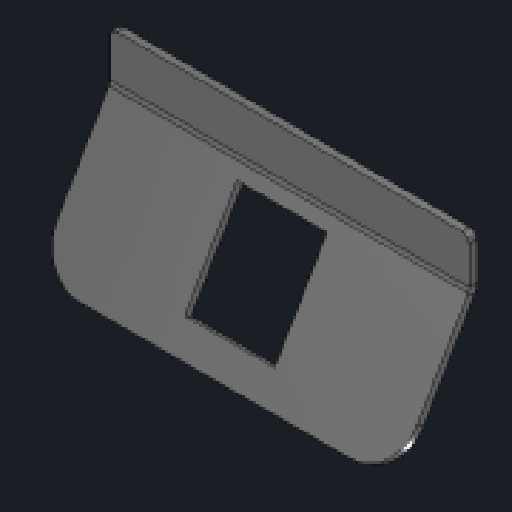
# Autodesk Inventor part: Model-4_Sheet Stifferner
Saved by Autodesk Inventor 2025.1 (Build 291241000, 241)
## iProperties
RuleStatus: InUse
Created: 2026-02-13
Part Number: Model-4_Sheet Stifferner
User Status: Released
Material: SS304
Document SubType Name: Sheet Metal
Designer: Desktop -24
Density: 7.99949 g/cm^3
Sheet Metal Rule: 1/4"
Appearance: Semi-Polished(1)
AfterDocNew0: Mat. Selection
encoded128: ÌSheet Metal (in)XÎ
Family: SS304
Author: Desktop -24
Revision Number: 0
Autodesk Inventor part; units mm, degrees
ref_plane "YZ Plane" through (0, 0, 0) normal (1, 0, 0) x (0, 1, 0)
ref_plane "XZ Plane" through (0, 0, 0) normal (0, 1, 0) x (-1, 0, 0)
ref_plane "XY Plane" through (0, 0, 0) normal (0, 0, 1) x (1, 0, 0)
sketch "Sketch1" plane through (0, 0, 0) normal (0, 0, 1) x (1, 0, 0)
  line L0 (-177.8, -19.05) -> (177.8, -19.05)
  line L1 (177.8, -19.05) -> (177.8, 19.05)
  line L2 (177.8, 19.05) -> (-177.8, 19.05)
  line L3 (-177.8, 19.05) -> (-177.8, -19.05)
  line L4 (-177.8, -19.05) -> (177.8, 19.05) construction
  line L5 (177.8, -19.05) -> (-177.8, 19.05) construction
  point P0 (0, 0)
  point P1 (0, 0)
  dimension "d31" = 355.6
  dimension "d32" = 38.1
  measures "d31" distance of L1.end L2.end
  measures "d32" distance of L0.end L1.end
extrude "Plate1" add sketch "Sketch1" along normal blind 6.35
sketch "Sketch3" plane through (177.8, -23.0251, 7.4151) normal (0, -0.5, -0.8660254) x (1, 0, 0)
  line L0 (-355.6, 0) -> (0, 0)
  line L1 (0, 0) -> (0, 125.3998)
  line L2 (0, 125.3998) -> (-355.6, 125.3998)
  line L3 (-355.6, 125.3998) -> (-355.6, 0)
  constraints: 6 end point, 1 horizontal, 1 perpendicular, 1 vertical
edge flange "Flange2" height 139.7 angle 30 thickness 6.35 bend radius 7.9502 thickness toward (0, -0.5, -0.8660254) relief tear relief width 6.35 relief depth 3.175 edges at (0, -19.05, 6.35) wall of the first edge with corners at (-177.8, -23.0251, 7.4151) (177.8, -23.0251, 7.4151) (177.8, -131.6245, 70.115) (-177.8, -131.6245, 70.115)
bend "Bend2"
corner "Corner2"
fillet "Corner Round1" radius 6.35 2 edges at (177.8, 19.05, 3.175) (-177.8, 19.05, 3.175)
fillet "Corner Round2" radius 38.1 2 edges at (177.8, -133.212, 67.3654) (-177.8, -133.212, 67.3654)
sketch "Sketch4" plane through (-177.8, -23.0251, 7.4151) normal (0, 0.5, 0.8660254) x (1, 0, 0)
  line L0 (152.4, -9.5123) -> (203.2, -9.5123)
  line L1 (215.9, -22.2123) -> (215.9, -85.7123)
  line L2 (203.2, -98.4123) -> (152.4, -98.4123)
  line L3 (139.7, -85.7123) -> (139.7, -22.2123)
  line L4 (139.7, -9.5123) -> (215.9, -98.4123) construction
  line L5 (215.9, -9.5123) -> (139.7, -98.4123) construction
  line L6 (38.1, -125.3998) -> (317.5, -125.3998) construction
  arc A0 (152.4, -9.5123) -> (139.7, -22.2123) centre (152.4, -22.2123) ccw
  arc A1 (215.9, -22.2123) -> (203.2, -9.5123) centre (203.2, -22.2123) ccw
  arc A2 (203.2, -98.4123) -> (215.9, -85.7123) centre (203.2, -85.7123) ccw
  arc A3 (139.7, -85.7123) -> (152.4, -98.4123) centre (152.4, -85.7123) ccw
  line L7 (63.5, -79.3623) -> (63.5, -28.5623) construction
  line L8 (50.8, -79.3623) -> (50.8, -28.5623)
  line L9 (76.2, -28.5623) -> (76.2, -79.3623)
  arc A4 (50.8, -79.3623) -> (76.2, -79.3623) centre (63.5, -79.3623) ccw
  arc A5 (76.2, -28.5623) -> (50.8, -28.5623) centre (63.5, -28.5623) ccw
  line L10 (0, -87.2998) -> (0, 0) projected
  line L11 (177.8, -53.9623) -> (177.8, -125.3998) construction
  line L12 (292.1, -79.3623) -> (292.1, -28.5623) construction
  line L13 (304.8, -79.3623) -> (304.8, -28.5623)
  line L14 (279.4, -28.5623) -> (279.4, -79.3623)
  arc A6 (279.4, -79.3623) -> (304.8, -79.3623) centre (292.1, -79.3623) ccw
  arc A7 (304.8, -28.5623) -> (279.4, -28.5623) centre (292.1, -28.5623) ccw
  point P0 (63.5, -53.9623)
  dimension "d45" = 26.9875
  dimension "d46" = 76.2
  dimension "d47" = 88.9
  dimension "d50" = 12.7
  dimension "d51" = 12.7
  dimension "d52" = 50.8
  dimension "d53" = 63.5
  dimension "d54" = 25.4
  constraints: 30 end point, 16 point on circle, 12 tangent, 8 centre point, 8 point on line, 6 symmetric about line, 4 midpoint, 3 parallel, 2 equal radius, 2 vertical, 1 horizontal, 1 horizontal alignment, 1 perpendicular, 1 vertical alignment, 2 other
  measures "d45" distance between parallel lines of L2 L6
  measures "d46" distance of L4.end L5.end
  measures "d47" distance of L5.end L4.start
  measures "d50" radius of A0
  measures "d51" radius of A1
  measures "d52" distance of L8.start L8.end
  measures "d53" distance between parallel lines of L10 L7
  measures "d54" distance between parallel lines of L9 L8
extrude "Cut1" cut sketch "Sketch4" against normal blind 6.35
equation "\"d48\" = Thickness"
equation "\"d15\" = Thickness"
equation "\"d33\" = BendReliefWidth"
equation "\"d34\" = BendReliefDepth"
equation "\"d35\" = MinimumRemnant"
equation "\"d36\" = TransitionRadius"
equation "\"d39\" = BendRadius"
equation "\"d40\" = CornerReliefSize"
equation "\"d41\" = GapSize"
equation "\"d42\" = JacobiRadiusSize"
equation "\"BendReliefWidth\" = Thickness"
equation "\"BendReliefDepth\" = 0.5 * Thickness"
equation "\"CornerReliefSize\" = 4 * Thickness"
equation "\"MinimumRemnant\" = 2 * Thickness"
equation "\"TransitionRadius\" = BendRadius"
equation "\"JacobiRadiusSize\" = Thickness"
equation "\"GapSize\" = Thickness"
equation "\"Thickness\" = 6.35"
equation "\"BendRadius\" = 7.9502"
body "Solid1"
